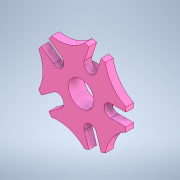
# Autodesk Inventor part: cruz de malta
Saved by Autodesk Inventor 2022 (Build 260153000, 153)
## iProperties
Created: 2023-03-13
Part Number: cruz de malta
Material: Genérico
Document SubType Name: Modeling
Designer: jpjoa
Density: 1 g/cm^3
Appearance: Rosa
Author: jpjoa
Autodesk Inventor part; units mm, degrees
ref_plane "YZ Plane" through (0, 0, 0) normal (1, 0, 0) x (0, 1, 0)
ref_plane "XZ Plane" through (0, 0, 0) normal (0, 1, 0) x (-1, 0, 0)
ref_plane "XY Plane" through (0, 0, 0) normal (0, 0, 1) x (1, 0, 0)
sketch "Esboço1" plane through (0, 0, 0) normal (0, 0, 1) x (1, 0, 0)
  circle A0 centre (0, 0) radius 50
  dimension "d9" = 100
  constraints: 1 centre point, 1 coincident
  measures "d9" diameter of A0
extrude "Extrusão1" add sketch "Esboço1" along normal blind 6
sketch "Esboço2" plane through (0, 0, 6) normal (0, 0, 1) x (1, 0, 0)
  line L0 (35, 50) -> (65, 50)
  line L1 (65, 50) -> (65, -50)
  line L2 (65, -50) -> (35, -50)
  line L3 (35, -50) -> (35, 50)
  line L4 (18, 5) -> (35, 5)
  line L5 (35, 5) -> (35, -5)
  line L6 (35, -5) -> (18, -5)
  line L7 (18, -5) -> (18, 5)
  point P0 (0, 0)
  point P1 (35, 0)
  point P2 (35, 0)
  point P3 (18, 0)
  dimension "d12" = 35
  dimension "d13" = 100
  dimension "d14" = 30
  dimension "d15" = 10
  dimension "d16" = 18
  constraints: 16 end point, 4 parallel, 3 midpoint, 2 horizontal, 2 horizontal alignment, 2 perpendicular, 1 coincident
  measures "d12" distance of point (35, 0) point (0, 0)
  measures "d13" distance between parallel lines of L2 L0
  measures "d14" distance between parallel lines of L1 L3
  measures "d15" distance between parallel lines of L6 L4
  measures "d16" distance from line of L7 point (0, 0)
extrude "Extrusão2" cut sketch "Esboço2" against normal through all
fillet "Arredondamento1" radius 5 2 edges at (18, -5, 3) (18, 5, 3)
pattern_circular "Padrão circular1" count 5 over 360 about axis through (0, 0, 0) along (0, 0, 1) of "Extrusão2", "Arredondamento1"
sketch "Esboço3" plane through (0, 0, 6) normal (0, 0, 1) x (1, 0, 0)
  circle A0 centre (0, 0) radius 10
  dimension "d23" = 20
  constraints: 1 centre point, 1 coincident
  measures "d23" diameter of A0
extrude "Extrusão3" cut sketch "Esboço3" against normal through all
sketch "Esboço4" plane through (0, 0, 6) normal (0, 0, 1) x (1, 0, 0)
  circle A0 centre (-60, 0) radius 30
  point P0 (0, 0)
  dimension "d26" = 60
  dimension "d27" = 60
  constraints: 1 centre point, 1 horizontal alignment
  measures "d26" diameter of A0
  measures "d27" distance of point (0, 0) A0.centre
extrude "Extrusão4" cut sketch "Esboço4" against normal through all
pattern_circular "Padrão circular2" count 5 over 360 about axis through (0, 0, 6) along (0, 0, -1) of "Extrusão4"
sketch "Esboço5" plane through (0, 0, 0) normal (0, 0, -1) x (-1, 0, 0)
  circle A0 centre (0, 0) radius 10 projected
  circle A1 centre (0, 0) radius 10 projected
  circle A2 centre (0, 0) radius 15
  dimension "d33" = 30
  constraints: 1 centre point, 1 coincident
  measures "d33" diameter of A2
extrude "Extrusão5" add sketch "Esboço5" along normal blind 6
